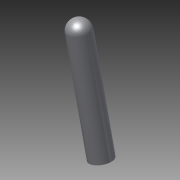
# Autodesk Inventor part: M20S-toggles
Saved by Autodesk Inventor 2015 SP1 (Build 190203100, 203)
## iProperties
Category: PARTsolutions
Company: NKKSWITCHES
Created: 2013-12-29
Part Number: M20S-toggles
Catalog Web Link: www.cadenas.de
Description: Bushing Mount Miniature Toggles - toggles-Series M - Miniature Toggles
Vendor: NKKSWITCHES
Document SubType Name: Modeling
Designer: PARTuser1
Manufacturer: NKKSWITCHES
Density: 1 g/cm^3
Material: Generic
Appearance: RGB(192.00000375509219,192.00000375509219,192.00000375509219)
PSOL_IDENT_0: {$CADENAS_DATA\23d-libs\nkkswitches\toggle\m\parts\m_bt_toggle.prj},215 {VTYP=3D},{NB=M20S-toggles},
PSOL_IDENT_1: {LINA=M20S-toggles},{NN=Bushing Mount Miniature Toggles - toggles},{DATE=28.05.2013 12:02:29},{GEOMD
PSOL_IDENT_2: ATE=28.05.2013 14:02:00},{VERSION=},{LINEID=10},{LINESUBID=-1},{WBVAR=TGGLS,CPS,CCLR}  {NB=M20S-togg
PSOL_IDENT_3: les},{LINA=M20S-toggles},{KT=DUMMY},{PN=M20S},{SRS=M20},{TGGLSALG='S', 'S - .413\" (10.5mm) Bat','S2
PSOL_IDENT_4: ', 'S2 - .200\" (5.08mm) Bat','S3', 'S3 - .256\" (6.5mm) Bat','E', 'E - .450\" (11.4mm) Flatted','E2
PSOL_IDENT_5: ', 'E2 - .256\" (6.5mm) Flatted','E4', 'E4 - .840\" (21.3mm) Flatted','Q', 'Q - .550\" (14.0mm) Cone
PSOL_IDENT_6: ','Q2', 'Q2 - .640\" (16.26mm) Cone','Q4', 'Q4 - .840\" (21.3mm) Cone','C', 'C - .571\" (14.5mm) Col
PSOL_IDENT_7: or Tipped Cone','D', 'D - .840\" (21.3mm) Color Tipped Cone','K1', 'K1 - .370\" (9.4mm) Paddle','K2'
PSOL_IDENT_8: , 'K2 - .559\" (14.2mm) Paddle','B', 'B - .453\" (11.5mm) Large Bat','B2', 'B2 - .689\" (17.5mm) Lar
PSOL_IDENT_9: ge Bat','R', 'R - .610\" (15.5mm) Large Flatted','L', 'L - .201\" (5.1mm) Dia. Locking Lever'},{TGGL
PSOL_IDENT_10: S=S},{CPSALG='','w/o Cap','B', 'B - For S Bat Toggle','C', 'C - Conical Cap for S Bat Toggle'},{CPS=
PSOL_IDENT_11: },{CPSPN=},{CCLRALG='','N/A'},{CCLR=},{DSH=},{HEIGHT=0.413},{SHEIGHT=0.0875},{ROTALG=0.23},{CPCAP=0.
PSOL_IDENT_12: 781525}
CNS_NN: Bushing Mount Miniature Toggles - toggles
CNS_NT: Series M - Miniature Toggles
CNS_NB: M20S-toggles
CNS_NBSYN: $PN.-toggles
CNS_LINA: M20S-toggles
CNS_PN: M20S
CNS_SRS: M20
CNS_TGGLSALG: 'S', 'S - .413" (10.5mm) Bat','S2', 'S2 - .200" (5.08mm) Bat','S3', 'S3 - .256" (6.5mm) Bat','E', 'E - .450" (11.4mm) Flatted','E2', 'E2 - .256" (6.5mm) Flatted','E4', 'E4 - .840" (21.3mm) Flatted','Q', 'Q - .550" (14.0mm) Cone','Q2', 'Q2 - .640" (16.26mm) Cone','Q4', 'Q4 - .840" (21.3mm) Cone','C', 'C - .571" (14.5mm) Color Tipped Cone','D', 'D - .840" (21.3mm) Color Tipped Cone','K1', 'K1 - .370" (9.4mm) Paddle','K2', 'K2 - .559" (14.2mm) Paddle','B', 'B - .453" (11.5mm) Large Bat','B2', 'B2 - .689" (17.5mm) Large Bat','R', 'R - .610" (15.5mm) Large Flatted','L', 'L - .201" (5.1mm) Dia. Locking Lever'
CNS_TGGLS: S - .413" (10.5mm) Bat
CNS_CPSALG: '','w/o Cap','B', 'B - For S Bat Toggle','C', 'C - Conical Cap for S Bat Toggle'
CNS_CPS: w/o Cap
CNS_CCLRALG: '','N/A'
CNS_CCLR: N/A
CNS_HEIGHT: 0.413
CNS_SHEIGHT: 0.087
CNS_ROTALG: 0.230
CNS_CPCAP: 0.782
SUPPLIER: NKKSWITCHES
ARTICLENO: M20S-toggles
BOMINFO: M20S-toggles
CREATOR: CADENAS GmbH
Title: M20S-toggles
Author: Cadenas PARTsolutions
Comments: Series M - Miniature Toggles
Autodesk Inventor part; units mm, degrees
sketch "Sketch_1" plane through (0, 0, 0) normal (0, 0, 1) x (1, 0, 0)
  line L0 (0.481, -4.3923) -> (-2.811, 10.4571)
  arc A0 (-1.1447, 9.3956) -> (-2.811, 10.4571) centre (-2.5086, 9.0932) ccw
  line L1 (-1.1447, 9.3956) -> (1.8449, -4.09)
  line L2 (1.8449, -4.09) -> (0.481, -4.3923)
  line L3 (0.481, -4.3923) -> (-2.811, 10.4571)
  constraints: 8 end point, 2 point on circle, 1 centre point
revolve "Revolution1" add sketch "Sketch_1" angle 360 about axis through (0.481, -4.3923, 0) along (0.2164396, -0.976296, 0)
ref_plane "rot_XY" through (0, -2.2225, 0) normal (0, 0, 1) x (1, 0, 0)
ref_plane "rot_YZ" through (0, -2.2225, 0) normal (1, 0, 0) x (0, 1, 0)
ref_plane "rot_ZX" through (0, -2.2225, 0) normal (0, 1, 0) x (0, 0, 1)
ref_plane "to_cap_XY" through (0, -2.2225, 0) normal (0, 1, 0) x (1, 0, 0)
ref_plane "to_cap_YZ" through (0, -2.2225, 0) normal (1, 0, 0) x (0, 0, -1)
ref_plane "to_cap_ZX" through (0, -2.2225, 0) normal (0, 0, -1) x (0, 1, 0)
body "Solid1"
